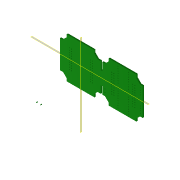
# Autodesk Inventor part: UC2_Insert_Feather_v3.brd_Kontur
Saved by Autodesk Inventor 2022 (Build 260153000, 153)
## iProperties
Created: 2022-01-18
Part Number: UC2_Insert_Feather_v3.brd_Kontur
Material: Generisch
Document SubType Name: Modeling
Designer: diederichbenedict
Density: 1 g/cm^3
Appearance: Board-Kontur
Author: diederichbenedict
Autodesk Inventor part; units mm, degrees
ref_plane "YZ Plane" through (0, 0, 0) normal (1, 0, 0) x (0, 1, 0)
ref_plane "XZ Plane" through (0, 0, 0) normal (0, 1, 0) x (-1, 0, 0)
ref_plane "XY Plane" through (0, 0, 0) normal (0, 0, 1) x (1, 0, 0)
sketch "Skizze1" plane through (0, 0, 0) normal (0, 0, 1) x (1, 0, 0)
  line L0 (-3.81, 37.465) -> (-3.81, 3.81)
  line L1 (-3.81, 3.81) -> (0, 3.81)
  line L2 (0, 3.81) -> (4.445, -0.635)
  line L3 (4.445, -0.635) -> (4.445, -3.81)
  line L4 (4.445, -3.81) -> (38.1, -3.81)
  line L5 (38.1, -3.81) -> (38.1, 0)
  line L6 (38.1, 0) -> (41.91, 3.81)
  line L7 (41.91, 3.81) -> (45.72, 3.81)
  line L8 (45.72, 3.81) -> (45.72, 12.7)
  line L9 (45.72, 12.7) -> (47.625, 12.7)
  line L10 (47.625, 12.7) -> (47.625, 3.81)
  line L11 (47.625, 3.81) -> (50.8, 3.81)
  line L12 (50.8, 3.81) -> (55.245, -0.635)
  line L13 (55.245, -0.635) -> (55.245, -3.81)
  line L14 (55.245, -3.81) -> (88.9, -3.81)
  line L15 (88.9, -3.81) -> (88.9, -0.635)
  line L16 (88.9, -0.635) -> (93.345, 3.81)
  line L17 (93.345, 3.81) -> (96.52, 3.81)
  line L18 (96.52, 3.81) -> (96.52, 37.465)
  line L19 (96.52, 37.465) -> (93.345, 37.465)
  line L20 (93.345, 37.465) -> (88.9, 41.91)
  line L21 (88.9, 41.91) -> (88.9, 45.72)
  line L22 (88.9, 45.72) -> (55.245, 45.72)
  line L23 (55.245, 45.72) -> (55.245, 42.545)
  line L24 (55.245, 42.545) -> (50.8, 38.1)
  line L25 (50.8, 38.1) -> (47.625, 38.1)
  line L26 (47.625, 38.1) -> (47.625, 28.575)
  line L27 (47.625, 28.575) -> (45.72, 28.575)
  line L28 (45.72, 28.575) -> (45.72, 38.1)
  line L29 (45.72, 38.1) -> (41.91, 38.1)
  line L30 (41.91, 38.1) -> (37.465, 42.545)
  line L31 (37.465, 42.545) -> (37.465, 45.72)
  line L32 (37.465, 45.72) -> (4.445, 45.72)
  line L33 (4.445, 45.72) -> (4.445, 42.545)
  line L34 (4.445, 42.545) -> (-0.635, 37.465)
  line L35 (-0.635, 37.465) -> (-3.81, 37.465)
  circle A0 centre (50.7, 11.28) radius 0.55
  circle A1 centre (50.7, 7.78) radius 0.55
  circle A2 centre (33.02, 27.94) radius 0.555
  circle A3 centre (7.62, 33.02) radius 0.555
  circle A4 centre (35.56, 33.02) radius 0.555
  circle A5 centre (7.62, 10.16) radius 0.555
  circle A6 centre (10.16, 25.4) radius 0.555
  circle A7 centre (35.56, 10.16) radius 0.555
  circle A8 centre (7.62, 25.4) radius 0.555
  circle A9 centre (7.62, 27.94) radius 0.555
  circle A10 centre (7.62, 22.86) radius 0.555
  circle A11 centre (33.02, 25.4) radius 0.555
  circle A12 centre (10.16, 22.86) radius 0.555
  circle A13 centre (10.16, 20.32) radius 0.555
  circle A14 centre (33.02, 17.78) radius 0.555
  circle A15 centre (33.02, 20.32) radius 0.555
  circle A16 centre (10.16, 17.78) radius 0.555
  circle A17 centre (10.16, 15.24) radius 0.555
  circle A18 centre (33.02, 22.86) radius 0.555
  circle A19 centre (7.62, 15.24) radius 0.555
  circle A20 centre (33.02, 15.24) radius 0.555
  circle A21 centre (7.62, 12.7) radius 0.555
  circle A22 centre (7.62, 17.78) radius 0.555
  circle A23 centre (35.56, 20.32) radius 0.555
  circle A24 centre (35.56, 22.86) radius 0.555
  circle A25 centre (35.56, 17.78) radius 0.555
  circle A26 centre (35.56, 12.7) radius 0.555
  circle A27 centre (35.56, 27.94) radius 0.555
  circle A28 centre (33.02, 10.16) radius 0.555
  circle A29 centre (10.16, 12.7) radius 0.555
  circle A30 centre (10.16, 33.02) radius 0.555
  circle A31 centre (7.62, 30.48) radius 0.555
  circle A32 centre (35.56, 30.48) radius 0.555
  circle A33 centre (33.02, 33.02) radius 0.555
  circle A34 centre (35.56, 15.24) radius 0.555
  circle A35 centre (33.02, 12.7) radius 0.555
  circle A36 centre (33.02, 30.48) radius 0.555
  circle A37 centre (10.16, 30.48) radius 0.555
  circle A38 centre (7.62, 20.32) radius 0.555
  circle A39 centre (35.56, 25.4) radius 0.555
  circle A40 centre (10.16, 10.16) radius 0.555
  circle A41 centre (10.16, 27.94) radius 0.555
  circle A42 centre (84.45, 27.94) radius 0.555
  circle A43 centre (59.05, 33.02) radius 0.555
  circle A44 centre (87, 33.02) radius 0.555
  circle A45 centre (59.05, 10.16) radius 0.555
  circle A46 centre (61.6, 25.4) radius 0.555
  circle A47 centre (87, 10.16) radius 0.555
  circle A48 centre (59.05, 25.4) radius 0.555
  circle A49 centre (59.05, 27.94) radius 0.555
  circle A50 centre (59.05, 22.86) radius 0.555
  circle A51 centre (84.45, 25.4) radius 0.555
  circle A52 centre (61.6, 22.86) radius 0.555
  circle A53 centre (61.6, 20.32) radius 0.555
  circle A54 centre (84.45, 17.78) radius 0.555
  circle A55 centre (84.45, 20.32) radius 0.555
  circle A56 centre (61.6, 17.78) radius 0.555
  circle A57 centre (61.6, 15.24) radius 0.555
  circle A58 centre (84.45, 22.86) radius 0.555
  circle A59 centre (59.05, 15.24) radius 0.555
  circle A60 centre (84.45, 15.24) radius 0.555
  circle A61 centre (59.05, 12.7) radius 0.555
  circle A62 centre (59.05, 17.78) radius 0.555
  circle A63 centre (87, 20.32) radius 0.555
  circle A64 centre (87, 22.86) radius 0.555
  circle A65 centre (87, 17.78) radius 0.555
  circle A66 centre (87, 12.7) radius 0.555
  circle A67 centre (87, 27.94) radius 0.555
  circle A68 centre (84.45, 10.16) radius 0.555
  circle A69 centre (61.6, 12.7) radius 0.555
  circle A70 centre (61.6, 33.02) radius 0.555
  circle A71 centre (59.05, 30.48) radius 0.555
  circle A72 centre (87, 30.48) radius 0.555
  circle A73 centre (84.45, 33.02) radius 0.555
  circle A74 centre (87, 15.24) radius 0.555
  circle A75 centre (84.45, 12.7) radius 0.555
  circle A76 centre (84.45, 30.48) radius 0.555
  circle A77 centre (61.6, 30.48) radius 0.555
  circle A78 centre (59.05, 20.32) radius 0.555
  circle A79 centre (87, 25.4) radius 0.555
  circle A80 centre (61.6, 10.16) radius 0.555
  circle A81 centre (61.6, 27.94) radius 0.555
  circle A82 centre (66.67, 17.14) radius 0.51
  circle A83 centre (66.67, 14.61) radius 0.51
  circle A84 centre (66.67, 12.07) radius 0.51
  circle A85 centre (66.67, 9.53) radius 0.51
  circle A86 centre (66.67, 6.99) radius 0.51
  circle A87 centre (66.67, 4.45) radius 0.51
  circle A88 centre (66.67, 1.91) radius 0.51
  circle A89 centre (66.67, -0.64) radius 0.51
  circle A90 centre (79.38, 17.14) radius 0.51
  circle A91 centre (79.38, 14.61) radius 0.51
  circle A92 centre (79.38, 12.07) radius 0.51
  circle A93 centre (79.38, 9.53) radius 0.51
  circle A94 centre (79.38, 6.99) radius 0.51
  circle A95 centre (79.38, 4.45) radius 0.51
  circle A96 centre (79.38, 1.91) radius 0.51
  circle A97 centre (79.38, -0.64) radius 0.51
  circle A98 centre (93.98, 15.24) radius 0.51
  circle A99 centre (93.98, 12.7) radius 0.51
  circle A100 centre (93.98, 10.16) radius 0.51
  circle A101 centre (93.98, 7.62) radius 0.51
  circle A102 centre (-32.38, -44.45) radius 0.405
  circle A103 centre (-27.3, -44.45) radius 0.405
  circle A104 centre (66.67, 43.18) radius 0.51
  circle A105 centre (66.67, 40.64) radius 0.51
  circle A106 centre (66.67, 38.1) radius 0.51
  circle A107 centre (66.67, 35.56) radius 0.51
  circle A108 centre (66.67, 33.02) radius 0.51
  circle A109 centre (66.67, 30.48) radius 0.51
  circle A110 centre (66.67, 27.94) radius 0.51
  circle A111 centre (66.67, 25.4) radius 0.51
  circle A112 centre (79.38, 43.18) radius 0.51
  circle A113 centre (79.38, 40.64) radius 0.51
  circle A114 centre (79.38, 38.1) radius 0.51
  circle A115 centre (79.38, 35.56) radius 0.51
  circle A116 centre (79.38, 33.02) radius 0.51
  circle A117 centre (79.38, 30.48) radius 0.51
  circle A118 centre (79.38, 27.94) radius 0.51
  circle A119 centre (79.38, 25.4) radius 0.51
  circle A120 centre (93.98, 34.29) radius 0.51
  circle A121 centre (93.98, 31.75) radius 0.51
  circle A122 centre (93.98, 29.21) radius 0.51
  circle A123 centre (93.98, 26.67) radius 0.51
  constraints: 124 centre point, 72 end point
extrude "UC2_Insert_Feather_v3.brd_Kontur" add sketch "Skizze1" along normal blind 1.6
ref_plane "Arbeitsebene1" through (4.445, 20.955, 0) normal (0, -1, 0) x (1, 0, 0)
ref_plane "Arbeitsebene2" through (20.955, 3.81, 0) normal (-1, 0, 0) x (0, 0, 1)
